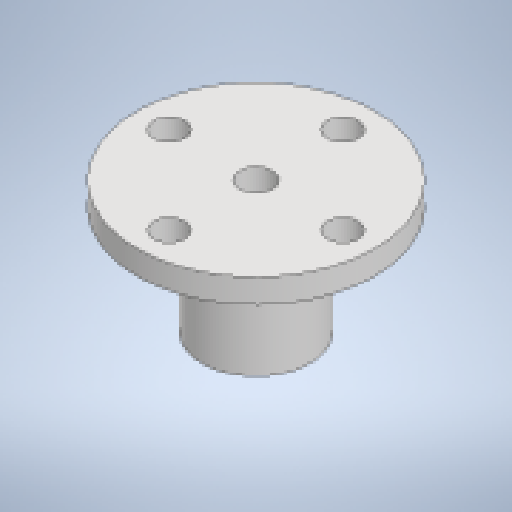
# Autodesk Inventor part: Acople motor
Saved by Autodesk Inventor 2024 (Build 280153000, 153)
## iProperties
Created: 2025-03-01
Part Number: Acople motor
Material: Genérico
Document SubType Name: Modeling
Designer: sergi
Density: 1 g/cm^3
Appearance: Valor por defecto
Author: sergi
Autodesk Inventor part; units mm, degrees
ref_plane "YZ Plane" through (0, 0, 0) normal (1, 0, 0) x (0, 1, 0)
ref_plane "XZ Plane" through (0, 0, 0) normal (0, 1, 0) x (-1, 0, 0)
ref_plane "XY Plane" through (0, 0, 0) normal (0, 0, 1) x (1, 0, 0)
sketch "Boceto1" plane through (0, 0, 0) normal (0, 1, 0) x (-1, 0, 0)
  circle A0 centre (0, 0) radius 5
  circle A1 centre (0, 0) radius 1.5
  dimension "d0" = 10
  dimension "d1" = 3
  constraints: 2 centre point, 2 coincident
  measures "d0" diameter of A0
  measures "d1" diameter of A1
extrude "Extrusión1" add sketch "Boceto1" along normal blind 10
sketch "Boceto2" plane through (0, 10, 0) normal (0, 1, 0) x (1, 0, 0)
  circle A0 centre (0, 0) radius 11
  circle A1 centre (0, 0) radius 5 projected
  circle A2 centre (0, 0) radius 1.5 projected
  dimension "d4" = 22
  constraints: 1 centre point, 1 coincident
  measures "d4" diameter of A0
extrude "Extrusión2" add sketch "Boceto2" along normal blind 2.2 contours A0 | A1
sketch "Boceto3" plane through (0, 12.2, 0) normal (0, 1, 0) x (1, 0, 0)
  circle A0 centre (0, 0) radius 9.475
  circle A1 centre (0, 0) radius 6.6
  line L0 (0, -6.6) -> (0, -9.475)
  circle A2 centre (0, -8.0375) radius 1.4375
  circle A3 centre (8.0375, 0) radius 1.4375
  circle A4 centre (0, 8.0375) radius 1.4375
  circle A5 centre (-8.0375, 0) radius 1.4375
  dimension "d7" = 18.95
  dimension "d8" = 13.2
  dimension "d11" = 360
  constraints: 4 centre point, 2 coincident, 2 end point, 2 vertical alignment, 1 midpoint, 13 other
hole "Agujero1" at (0, 12.2, 8.0375) at (-8.0375, 12.2, 0) at (0, 12.2, -8.0375) at (8.0375, 12.2, 0) direction (0, -1, 0) diameter 2.85 end through all
